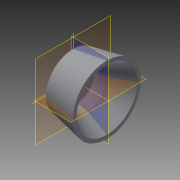
# Autodesk Inventor part: ScheinwerferFront
Saved by Autodesk Inventor 2015 (Build 190159000, 159)
## iProperties
Created: 2019-02-15
Part Number: ScheinwerferFront
Material: Generisch
Document SubType Name: Modeling
Designer: Boris
Density: 1 g/cm^3
Appearance: Vorgabe
Author: Boris
Autodesk Inventor part; units mm, degrees
sketch "Skizze1" plane through (0, 0, 0) normal (0, 0, 1) x (1, 0, 0)
  line L0 (5, 3.5) -> (0, 2.5)
  line L1 (5, 5.0297) -> (0, 4.0297)
  line L2 (0, 2.5) -> (0, 4.0297)
  line L3 (5, 5.0297) -> (5, 3.5)
  line L4 (-1, 0) -> (6, 0) projected
  point P0 (0, 0)
  dimension "d53" = 2.5
  dimension "d55" = 1.5
  constraints: 8 end point, 2 vertical, 1 parallel
  measures "d53" distance of point (0, 0) L0.end
  measures "d55" distance between parallel lines of L0 L1
revolve "Umdrehung1" add sketch "Skizze1" angle 360 about axis through (-10, 0, 0) along (1, 0, 0)
fillet "Rundung7" radius 1 1 edges at (0, -2.5, 0)
chamfer "Fase1" distance 3 distance2 1 1 edges at (5, -3.5, 0) measured on face at (4.5097, -3.4019, 0)
